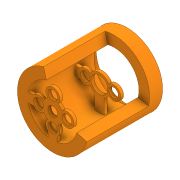
# Autodesk Inventor part: 3rd Axis
Saved by Autodesk Inventor 2020 (Build 240168000, 168)
## iProperties
Created: 2021-06-27
Part Number: 3rd Axis
Material: Generic
Document SubType Name: Modeling
Designer: Coy
Density: 1 g/cm^3
Appearance: Orange
Author: Coy
Autodesk Inventor part; units mm, degrees
ref_plane "YZ Plane" through (0, 0, 0) normal (1, 0, 0) x (0, 1, 0)
ref_plane "XZ Plane" through (0, 0, 0) normal (0, 1, 0) x (-1, 0, 0)
ref_plane "XY Plane" through (0, 0, 0) normal (0, 0, 1) x (1, 0, 0)
sketch "Sketch1" plane through (0, 0, 0) normal (0, 0, 1) x (1, 0, 0)
  circle A0 centre (0, 0) radius 30
  circle A1 centre (0, 0) radius 26
  dimension "d0" = 60
  dimension "d1" = 52
  constraints: 2 centre point, 2 coincident
  measures "d0" diameter of A0
  measures "d1" diameter of A1
extrude "Extrusion1" add sketch "Sketch1" along normal blind 7
sketch "Sketch2" plane through (0, 0, 7) normal (0, 0, 1) x (1, 0, 0)
  circle A0 centre (0, 0) radius 30 projected
  circle A1 centre (0, 0) radius 21
  dimension "d4" = 42
  constraints: 1 centre point, 1 coincident
  measures "d4" diameter of A1
extrude "Extrusion2" add sketch "Sketch2" along normal blind 14
chamfer "Chamfer1" distance 7 angle 2 1 edges at (-26, 0, 0) measured on face at (-26, 0, 0.5)
sketch "Sketch3" plane through (0, 0, 0) normal (0, 0, -1) x (-1, 0, 0)
  circle A0 centre (0, 0) radius 26 construction
  circle A1 centre (0, 0) radius 26.2444 projected
  arc A2 (-25.9992, -0.2) -> (-25.9992, 0.2) centre (-26, 0) ccw
  line L0 (-26.2437, -0.2019) -> (-25.9985, -0.2)
  line L1 (-26.2437, 0.2019) -> (-25.9985, 0.2)
  line L2 (-22.6267, -13.2967) -> (-22.4153, -13.1724)
  arc A3 (-22.416, -13.1728) -> (-22.616, -12.8264) centre (-22.5167, -13) ccw
  line L3 (-22.8286, -12.947) -> (-22.6153, -12.826)
  line L4 (-12.947, -22.8286) -> (-12.826, -22.6153)
  arc A4 (-12.8264, -22.616) -> (-13.1728, -22.416) centre (-13, -22.5167) ccw
  line L5 (-13.2967, -22.6267) -> (-13.1724, -22.4153)
  line L6 (0.2019, -26.2437) -> (0.2, -25.9985)
  arc A5 (0.2, -25.9992) -> (-0.2, -25.9992) centre (0, -26) ccw
  line L7 (-0.2019, -26.2437) -> (-0.2, -25.9985)
  line L8 (13.2967, -22.6267) -> (13.1724, -22.4153)
  arc A6 (13.1728, -22.416) -> (12.8264, -22.616) centre (13, -22.5167) ccw
  line L9 (12.947, -22.8286) -> (12.826, -22.6153)
  line L10 (22.8286, -12.947) -> (22.6153, -12.826)
  arc A7 (22.616, -12.8264) -> (22.416, -13.1728) centre (22.5167, -13) ccw
  line L11 (22.6267, -13.2967) -> (22.4153, -13.1724)
  line L12 (26.2437, 0.2019) -> (25.9985, 0.2)
  arc A8 (25.9992, 0.2) -> (25.9992, -0.2) centre (26, 0) ccw
  line L13 (26.2437, -0.2019) -> (25.9985, -0.2)
  line L14 (22.6267, 13.2967) -> (22.4153, 13.1724)
  arc A9 (22.416, 13.1728) -> (22.616, 12.8264) centre (22.5167, 13) ccw
  line L15 (22.8286, 12.947) -> (22.6153, 12.826)
  line L16 (12.947, 22.8286) -> (12.826, 22.6153)
  arc A10 (12.8264, 22.616) -> (13.1728, 22.416) centre (13, 22.5167) ccw
  line L17 (13.2967, 22.6267) -> (13.1724, 22.4153)
  line L18 (-0.2019, 26.2437) -> (-0.2, 25.9985)
  arc A11 (-0.2, 25.9992) -> (0.2, 25.9992) centre (0, 26) ccw
  line L19 (0.2019, 26.2437) -> (0.2, 25.9985)
  line L20 (-13.2967, 22.6267) -> (-13.1724, 22.4153)
  arc A12 (-13.1728, 22.416) -> (-12.8264, 22.616) centre (-13, 22.5167) ccw
  line L21 (-12.947, 22.8286) -> (-12.826, 22.6153)
  line L22 (-22.8286, 12.947) -> (-22.6153, 12.826)
  arc A13 (-22.616, 12.8264) -> (-22.416, 13.1728) centre (-22.5167, 13) ccw
  line L23 (-22.6267, 13.2967) -> (-22.4153, 13.1724)
  point P0 (0.2, 25.9992)
  point P1 (-12.8264, 22.616)
  point P2 (-25.9992, 0.2)
  point P3 (-25.9992, -0.2)
  point P4 (-22.616, -12.8264)
  point P5 (-0.2, -25.9992)
  point P6 (12.8264, -22.616)
  point P7 (25.9992, -0.2)
  point P8 (22.616, 12.8264)
  dimension "d10" = 0.4
  dimension "d13" = 360
  constraints: 53 point on circle, 48 end point, 12 centre point, 2 line through centre, 2 tangent, 122 other
  measures "d10" diameter of A2
extrude "Extrusion3" add sketch "Sketch3" against normal up to surface (7 mm away) contours A1 L13 A8 L12 | L15 A9 L14 A1 | A1 L11 A7 L10 | L17 A10 L16 A1 | A1 L9 A6 L8 | L19 A11 L18 A1 | A1 L7 A5 L6 | L21 A12 L20 A1 | A1 L5 A4 L4 | L23 A13 L22 A1 | A1 L3 A3 L2 | L1 A2 L0 A1
sketch "Sketch5" plane through (0, 0, 21) normal (0, 0, 1) x (1, 0, 0)
  circle A0 centre (0, 0) radius 7
  circle A1 centre (0, 0) radius 30 projected
  line L0 (-30, 0) -> (30, 0) construction
  circle A2 centre (12, 0) radius 4
  circle A3 centre (-12, 0) radius 4
  circle A4 centre (0, 0) radius 21 projected
  line L1 (-20.6155, 4) -> (-16.4721, 4)
  line L2 (-20.6155, -4) -> (-16.4721, -4)
  arc A5 (-16.4721, -4) -> (-7.875, -4.3571) centre (-12, 0) ccw
  arc A6 (-7.875, 4.3571) -> (-16.4721, 4) centre (-12, 0) ccw
  arc A7 (7.875, 4.3571) -> (-7.875, 4.3571) centre (0, 0) ccw
  arc A8 (7.875, -4.3571) -> (18, 0) centre (12, 0) ccw
  arc A9 (18, 0) -> (7.875, 4.3571) centre (12, 0) ccw
  line L3 (0, 0) -> (0, -21) construction
  line L4 (4, -8.0623) -> (4, -20.6155)
  line L5 (-4, -8.0623) -> (-4, -20.6155)
  arc A10 (-7.875, -4.3571) -> (-4, -8.0623) centre (0, 0) ccw
  arc A11 (4, -8.0623) -> (7.875, -4.3571) centre (0, 0) ccw
  point P0 (20.6155, 4)
  point P1 (20.6155, -4)
  point P2 (16.4721, 4)
  point P3 (16.4721, -4)
  dimension "d17" = 14
  dimension "d19" = 8
  dimension "d20" = 8
  dimension "d21" = 12
  dimension "d22" = 12
  dimension "d28" = 4
  dimension "d29" = 4
  constraints: 18 point on circle, 12 end point, 10 centre point, 3 horizontal, 3 point on line, 2 parallel, 2 tangent, 1 coincident, 1 vertical, 8 other
  measures "d17" diameter of A0
  measures "d19" diameter of A2
  measures "d20" diameter of A3
  measures "d21" distance of point (0, 0) A2.centre
  measures "d22" distance of point (0, 0) A3.centre
  measures "d28" distance between parallel lines of L3 L4
  measures "d29" distance between parallel lines of L3 L5
extrude "Extrusion4" add sketch "Sketch5" along normal blind 2.5 contours A1 | L1 A6 A7 A9 A8 A11 L4 A4 L5 A10 A5 L2
sketch "Sketch6" plane through (0, 0, 23.5) normal (0, 0, 1) x (1, 0, 0)
  line L0 (0, 0) -> (-7.7646, 28.9778)
  circle A0 centre (0, 0) radius 30 projected
  line L1 (0, 0) -> (28.9778, -7.7646)
  line L2 (0, 0) -> (0, 36.0418) construction
  circle A1 centre (0, 0) radius 30 projected
  arc A2 (4, -8.0623) -> (7.875, -4.3571) centre (0, 0) ccw projected
  arc A3 (7.875, -4.3571) -> (7.875, 4.3571) centre (12, 0) ccw projected
  arc A4 (7.875, 4.3571) -> (-7.875, 4.3571) centre (0, 0) ccw projected
  arc A5 (-7.875, 4.3571) -> (-16.4721, 4) centre (-12, 0) ccw projected
  line L3 (-16.4721, 4) -> (-20.6155, 4) projected
  arc A6 (4, -20.6155) -> (-20.6155, 4) centre (0, 0) ccw projected
  line L4 (4, -20.6155) -> (4, -8.0623) projected
  circle A7 centre (0, 0) radius 7 projected
  circle A8 centre (-12, 0) radius 4 projected
  circle A9 centre (12, 0) radius 4 projected
  arc A10 (-7.875, -4.3571) -> (-4, -8.0623) centre (0, 0) ccw projected
  line L5 (-4, -8.0623) -> (-4, -20.6155) projected
  arc A11 (-20.6155, -4) -> (-4, -20.6155) centre (0, 0) ccw projected
  line L6 (-20.6155, -4) -> (-16.4721, -4) projected
  arc A12 (-16.4721, -4) -> (-7.875, -4.3571) centre (-12, 0) ccw projected
  point P0 (-5.4352, 20.2844)
  point P1 (20.2844, -5.4352)
  dimension "d30" = 120
  dimension "d31" = 15
  constraints: 6 end point, 2 point on circle, 1 vertical
  measures "d30" angle of L1 L0
  measures "d31" angle of L2 L0
extrude "Extrusion5" cut sketch "Sketch6" against normal blind 12.5 contours L0 A0 L1 A6
sketch "Sketch7" plane through (0, 0, 23.5) normal (0, 0, 1) x (1, 0, 0)
  line L0 (28.9778, -7.7646) -> (20.2844, -5.4352) projected
  arc A0 (4, -20.6155) -> (20.2844, -5.4352) centre (0, 0) ccw projected
  line L1 (4, -20.6155) -> (4, -8.0623) projected
  arc A1 (4, -8.0623) -> (7.875, -4.3571) centre (0, 0) ccw projected
  arc A2 (7.875, -4.3571) -> (7.875, 4.3571) centre (12, 0) ccw projected
  arc A3 (7.875, 4.3571) -> (-7.875, 4.3571) centre (0, 0) ccw projected
  arc A4 (-7.875, 4.3571) -> (-16.4721, 4) centre (-12, 0) ccw projected
  line L2 (-16.4721, 4) -> (-20.6155, 4) projected
  arc A5 (-5.4352, 20.2844) -> (-20.6155, 4) centre (0, 0) ccw projected
  line L3 (-5.4352, 20.2844) -> (-7.7646, 28.9778) projected
  arc A6 (-7.7646, 28.9778) -> (28.9778, -7.7646) centre (0, 0) ccw projected
  circle A7 centre (0, 0) radius 7 projected
  circle A8 centre (-12, 0) radius 4 projected
  circle A9 centre (12, 0) radius 4 projected
  arc A10 (-7.875, -4.3571) -> (-4, -8.0623) centre (0, 0) ccw projected
  line L4 (-4, -8.0623) -> (-4, -20.6155) projected
  arc A11 (-20.6155, -4) -> (-4, -20.6155) centre (0, 0) ccw projected
  line L5 (-20.6155, -4) -> (-16.4721, -4) projected
  arc A12 (-16.4721, -4) -> (-7.875, -4.3571) centre (-12, 0) ccw projected
  line L6 (28.9778, -7.7646) -> (20.2844, -5.4352) projected
  arc A13 (-5.4352, 20.2844) -> (20.2844, -5.4352) centre (0, 0) ccw
  point P0 (4, -20.6155)
  point P1 (-20.6155, -4)
  constraints: 2 end point, 2 point on circle, 1 centre point, 1 coincident
extrude "Extrusion6" add sketch "Sketch7" along normal blind 37 contours A6 L3 A5 A13 A11 A0 L0
sketch "Sketch8" plane through (0, 0, 60.5) normal (0, 0, 1) x (1, 0, 0)
  circle A0 centre (12, 0) radius 4 projected
  circle A1 centre (12, 0) radius 4
  circle A2 centre (0, 0) radius 7 projected
  circle A3 centre (0, 12) radius 4
  circle A4 centre (-12, 0) radius 4
  circle A5 centre (0, -12) radius 4
  arc A6 (-7.875, 4.3571) -> (-7.875, -4.3571) centre (-12, 0) ccw
  arc A7 (4.3571, 7.875) -> (-4.3571, 7.875) centre (0, 12) ccw
  arc A8 (7.875, -4.3571) -> (7.875, 4.3571) centre (12, 0) ccw
  arc A9 (-4.3571, -7.875) -> (4.3571, -7.875) centre (0, -12) ccw
  line L0 (-16.4721, 4) -> (-20.6155, 4) projected
  line L1 (-20.6155, -4) -> (-16.4721, -4) projected
  line L2 (-4, -8.0623) -> (-4, -20.6155) projected
  line L3 (4, -20.6155) -> (4, -8.0623) projected
  arc A10 (-7.875, -4.3571) -> (-4, -8.0623) centre (0, 0) ccw
  arc A11 (4, -8.0623) -> (7.875, -4.3571) centre (0, 0) ccw
  arc A12 (7.875, 4.3571) -> (4.3571, 7.875) centre (0, 0) ccw
  arc A13 (-4.3571, 7.875) -> (-7.875, 4.3571) centre (0, 0) ccw
  arc A14 (-5.4352, 20.2844) -> (20.2844, -5.4352) centre (0, 0) ccw projected
  arc A15 (-5.4352, 20.2844) -> (20.2844, -5.4352) centre (0, 0) ccw projected
  line L4 (-5.4352, 20.2844) -> (-7.7646, 28.9778) projected
  arc A16 (-7.7646, 28.9778) -> (28.9778, -7.7646) centre (0, 0) ccw projected
  line L5 (28.9778, -7.7646) -> (20.2844, -5.4352) projected
  circle A17 centre (0, 0) radius 7 projected
  circle A18 centre (0, 0) radius 4
  point P0 (-4, -16.4721)
  point P1 (4, -16.4721)
  point P2 (20.2844, -5.4352)
  dimension "d38" = 360
  dimension "d40" = 2
  dimension "d41" = 2
  dimension "d42" = 2
  dimension "d43" = 2
  dimension "d47" = 8
  constraints: 18 point on circle, 13 centre point, 2 coincident, 2 point on line, 9 other
  measures "d40" radial gap between concentric circles of A4 A6
  measures "d41" radial gap between concentric circles of A3 A7
  measures "d42" radial gap between concentric circles of A0 A8
  measures "d43" radial gap between concentric circles of A5 A9
  measures "d47" diameter of A18
extrude "Extrusion7" add sketch "Sketch8" along normal blind 2.5 contours A2 | L3 A9 L2 A5 | A5 L2 A10 A6 A13 A7 A12 A8 A11 L3 | L3 A11 A9 | L2 A9 A10 | L3 A14 L2 A9 | A14 L5 A16 L4 | A14 L0 A6 L1
body "Solid1"
